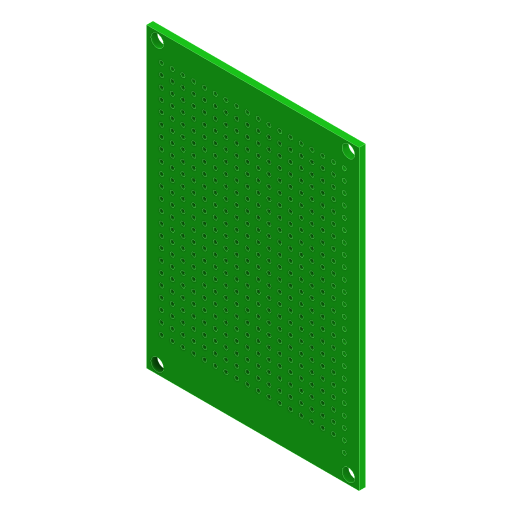
# Autodesk Inventor part: Плата главная
Saved by Autodesk Inventor 2023 (Build 270158000, 158)
## iProperties
Created: 2023-01-03
Part Number: Плата главная
Material: Типовые
Document SubType Name: Modeling
Designer: Admin
Density: 1 g/cm^3
Appearance: По умолчанию
Author: Admin
Autodesk Inventor part; units mm, degrees
ref_plane "YZ Plane" through (0, 0, 0) normal (1, 0, 0) x (0, 1, 0)
ref_plane "XZ Plane" through (0, 0, 0) normal (0, 1, 0) x (-1, 0, 0)
ref_plane "XY Plane" through (0, 0, 0) normal (0, 0, 1) x (1, 0, 0)
sketch "Эскиз1" plane through (0, 0, 0) normal (0, 0, 1) x (1, 0, 0)
  line L0 (25, 35) -> (-25, 35)
  line L1 (-25, 35) -> (-25, -35)
  line L2 (-25, -35) -> (25, -35)
  line L3 (25, -35) -> (25, 35)
  circle A0 centre (22.5, 33) radius 1.5
  circle A1 centre (-22.5, 33) radius 1.5
  circle A2 centre (-22.5, -33) radius 1.5
  circle A3 centre (22.5, -33) radius 1.5
  line L4 (0, 0) -> (8.4317, 0) construction
  line L5 (8.4317, 0) -> (0, 0) construction
  line L6 (0, 0) -> (0, -9.142) construction
  circle A4 centre (21.505, -28.98) radius 0.5
  circle A5 centre (21.505, -26.46) radius 0.5
  circle A6 centre (21.505, -23.94) radius 0.5
  circle A7 centre (21.505, -21.42) radius 0.5
  circle A8 centre (21.505, -18.9) radius 0.5
  circle A9 centre (21.505, -16.38) radius 0.5
  circle A10 centre (21.505, -13.86) radius 0.5
  circle A11 centre (21.505, -11.34) radius 0.5
  circle A12 centre (21.505, -8.82) radius 0.5
  circle A13 centre (21.505, -6.3) radius 0.5
  circle A14 centre (21.505, -3.78) radius 0.5
  circle A15 centre (21.505, -1.26) radius 0.5
  circle A16 centre (21.505, 1.26) radius 0.5
  circle A17 centre (21.505, 3.78) radius 0.5
  circle A18 centre (21.505, 6.3) radius 0.5
  circle A19 centre (21.505, 8.82) radius 0.5
  circle A20 centre (21.505, 11.34) radius 0.5
  circle A21 centre (21.505, 13.86) radius 0.5
  circle A22 centre (21.505, 16.38) radius 0.5
  circle A23 centre (21.505, 18.9) radius 0.5
  circle A24 centre (21.505, 21.42) radius 0.5
  circle A25 centre (21.505, 23.94) radius 0.5
  circle A26 centre (21.505, 26.46) radius 0.5
  circle A27 centre (21.505, 28.98) radius 0.5
  line L7 (25, 0) -> (23.0544, 0) construction
  circle A28 centre (18.975, -26.46) radius 0.5
  circle A29 centre (18.975, -23.94) radius 0.5
  circle A30 centre (18.975, -21.42) radius 0.5
  circle A31 centre (18.975, -18.9) radius 0.5
  circle A32 centre (18.975, -16.38) radius 0.5
  circle A33 centre (18.975, -13.86) radius 0.5
  circle A34 centre (18.975, -11.34) radius 0.5
  circle A35 centre (18.975, -8.82) radius 0.5
  circle A36 centre (18.975, -6.3) radius 0.5
  circle A37 centre (18.975, -3.78) radius 0.5
  circle A38 centre (18.975, -1.26) radius 0.5
  circle A39 centre (18.975, 1.26) radius 0.5
  circle A40 centre (18.975, 3.78) radius 0.5
  circle A41 centre (18.975, 6.3) radius 0.5
  circle A42 centre (18.975, 8.82) radius 0.5
  circle A43 centre (18.975, 11.34) radius 0.5
  circle A44 centre (18.975, 13.86) radius 0.5
  circle A45 centre (18.975, 16.38) radius 0.5
  circle A46 centre (18.975, 18.9) radius 0.5
  circle A47 centre (18.975, 21.42) radius 0.5
  circle A48 centre (18.975, 23.94) radius 0.5
  circle A49 centre (18.975, 26.46) radius 0.5
  circle A50 centre (18.975, 28.98) radius 0.5
  circle A51 centre (16.445, -26.46) radius 0.5
  circle A52 centre (16.445, -23.94) radius 0.5
  circle A53 centre (16.445, -21.42) radius 0.5
  circle A54 centre (16.445, -18.9) radius 0.5
  circle A55 centre (16.445, -16.38) radius 0.5
  circle A56 centre (16.445, -13.86) radius 0.5
  circle A57 centre (16.445, -11.34) radius 0.5
  circle A58 centre (16.445, -8.82) radius 0.5
  circle A59 centre (16.445, -6.3) radius 0.5
  circle A60 centre (16.445, -3.78) radius 0.5
  circle A61 centre (16.445, -1.26) radius 0.5
  circle A62 centre (16.445, 1.26) radius 0.5
  circle A63 centre (16.445, 3.78) radius 0.5
  circle A64 centre (16.445, 6.3) radius 0.5
  circle A65 centre (16.445, 8.82) radius 0.5
  circle A66 centre (16.445, 11.34) radius 0.5
  circle A67 centre (16.445, 13.86) radius 0.5
  circle A68 centre (16.445, 16.38) radius 0.5
  circle A69 centre (16.445, 18.9) radius 0.5
  circle A70 centre (16.445, 21.42) radius 0.5
  circle A71 centre (16.445, 23.94) radius 0.5
  circle A72 centre (16.445, 26.46) radius 0.5
  circle A73 centre (16.445, 28.98) radius 0.5
  circle A74 centre (13.915, -26.46) radius 0.5
  circle A75 centre (13.915, -23.94) radius 0.5
  circle A76 centre (13.915, -21.42) radius 0.5
  circle A77 centre (13.915, -18.9) radius 0.5
  circle A78 centre (13.915, -16.38) radius 0.5
  circle A79 centre (13.915, -13.86) radius 0.5
  circle A80 centre (13.915, -11.34) radius 0.5
  circle A81 centre (13.915, -8.82) radius 0.5
  circle A82 centre (13.915, -6.3) radius 0.5
  circle A83 centre (13.915, -3.78) radius 0.5
  circle A84 centre (13.915, -1.26) radius 0.5
  circle A85 centre (13.915, 1.26) radius 0.5
  circle A86 centre (13.915, 3.78) radius 0.5
  circle A87 centre (13.915, 6.3) radius 0.5
  circle A88 centre (13.915, 8.82) radius 0.5
  circle A89 centre (13.915, 11.34) radius 0.5
  circle A90 centre (13.915, 13.86) radius 0.5
  circle A91 centre (13.915, 16.38) radius 0.5
  circle A92 centre (13.915, 18.9) radius 0.5
  circle A93 centre (13.915, 21.42) radius 0.5
  circle A94 centre (13.915, 23.94) radius 0.5
  circle A95 centre (13.915, 26.46) radius 0.5
  circle A96 centre (13.915, 28.98) radius 0.5
  circle A97 centre (11.385, -26.46) radius 0.5
  circle A98 centre (11.385, -23.94) radius 0.5
  circle A99 centre (11.385, -21.42) radius 0.5
  circle A100 centre (11.385, -18.9) radius 0.5
  circle A101 centre (11.385, -16.38) radius 0.5
  circle A102 centre (11.385, -13.86) radius 0.5
  circle A103 centre (11.385, -11.34) radius 0.5
  circle A104 centre (11.385, -8.82) radius 0.5
  circle A105 centre (11.385, -6.3) radius 0.5
  circle A106 centre (11.385, -3.78) radius 0.5
  circle A107 centre (11.385, -1.26) radius 0.5
  circle A108 centre (11.385, 1.26) radius 0.5
  circle A109 centre (11.385, 3.78) radius 0.5
  circle A110 centre (11.385, 6.3) radius 0.5
  circle A111 centre (11.385, 8.82) radius 0.5
  circle A112 centre (11.385, 11.34) radius 0.5
  circle A113 centre (11.385, 13.86) radius 0.5
  circle A114 centre (11.385, 16.38) radius 0.5
  circle A115 centre (11.385, 18.9) radius 0.5
  circle A116 centre (11.385, 21.42) radius 0.5
  circle A117 centre (11.385, 23.94) radius 0.5
  circle A118 centre (11.385, 26.46) radius 0.5
  circle A119 centre (11.385, 28.98) radius 0.5
  circle A120 centre (8.855, -26.46) radius 0.5
  circle A121 centre (8.855, -23.94) radius 0.5
  circle A122 centre (8.855, -21.42) radius 0.5
  circle A123 centre (8.855, -18.9) radius 0.5
  circle A124 centre (8.855, -16.38) radius 0.5
  circle A125 centre (8.855, -13.86) radius 0.5
  circle A126 centre (8.855, -11.34) radius 0.5
  circle A127 centre (8.855, -8.82) radius 0.5
  circle A128 centre (8.855, -6.3) radius 0.5
  circle A129 centre (8.855, -3.78) radius 0.5
  circle A130 centre (8.855, -1.26) radius 0.5
  circle A131 centre (8.855, 1.26) radius 0.5
  circle A132 centre (8.855, 3.78) radius 0.5
  circle A133 centre (8.855, 6.3) radius 0.5
  circle A134 centre (8.855, 8.82) radius 0.5
  circle A135 centre (8.855, 11.34) radius 0.5
  circle A136 centre (8.855, 13.86) radius 0.5
  circle A137 centre (8.855, 16.38) radius 0.5
  circle A138 centre (8.855, 18.9) radius 0.5
  circle A139 centre (8.855, 21.42) radius 0.5
  circle A140 centre (8.855, 23.94) radius 0.5
  circle A141 centre (8.855, 26.46) radius 0.5
  circle A142 centre (8.855, 28.98) radius 0.5
  circle A143 centre (6.325, -26.46) radius 0.5
  circle A144 centre (6.325, -23.94) radius 0.5
  circle A145 centre (6.325, -21.42) radius 0.5
  circle A146 centre (6.325, -18.9) radius 0.5
  circle A147 centre (6.325, -16.38) radius 0.5
  circle A148 centre (6.325, -13.86) radius 0.5
  circle A149 centre (6.325, -11.34) radius 0.5
  circle A150 centre (6.325, -8.82) radius 0.5
  circle A151 centre (6.325, -6.3) radius 0.5
  circle A152 centre (6.325, -3.78) radius 0.5
  circle A153 centre (6.325, -1.26) radius 0.5
  circle A154 centre (6.325, 1.26) radius 0.5
  circle A155 centre (6.325, 3.78) radius 0.5
  circle A156 centre (6.325, 6.3) radius 0.5
  circle A157 centre (6.325, 8.82) radius 0.5
  circle A158 centre (6.325, 11.34) radius 0.5
  circle A159 centre (6.325, 13.86) radius 0.5
  circle A160 centre (6.325, 16.38) radius 0.5
  circle A161 centre (6.325, 18.9) radius 0.5
  circle A162 centre (6.325, 21.42) radius 0.5
  circle A163 centre (6.325, 23.94) radius 0.5
  circle A164 centre (6.325, 26.46) radius 0.5
  circle A165 centre (6.325, 28.98) radius 0.5
  circle A166 centre (3.795, -26.46) radius 0.5
  circle A167 centre (3.795, -23.94) radius 0.5
  circle A168 centre (3.795, -21.42) radius 0.5
  circle A169 centre (3.795, -18.9) radius 0.5
  circle A170 centre (3.795, -16.38) radius 0.5
  circle A171 centre (3.795, -13.86) radius 0.5
  circle A172 centre (3.795, -11.34) radius 0.5
  circle A173 centre (3.795, -8.82) radius 0.5
  circle A174 centre (3.795, -6.3) radius 0.5
  circle A175 centre (3.795, -3.78) radius 0.5
  circle A176 centre (3.795, -1.26) radius 0.5
  circle A177 centre (3.795, 1.26) radius 0.5
  circle A178 centre (3.795, 3.78) radius 0.5
  circle A179 centre (3.795, 6.3) radius 0.5
  circle A180 centre (3.795, 8.82) radius 0.5
  circle A181 centre (3.795, 11.34) radius 0.5
  circle A182 centre (3.795, 13.86) radius 0.5
  circle A183 centre (3.795, 16.38) radius 0.5
  circle A184 centre (3.795, 18.9) radius 0.5
  circle A185 centre (3.795, 21.42) radius 0.5
  circle A186 centre (3.795, 23.94) radius 0.5
  circle A187 centre (3.795, 26.46) radius 0.5
  circle A188 centre (3.795, 28.98) radius 0.5
  circle A189 centre (1.265, -26.46) radius 0.5
  circle A190 centre (1.265, -23.94) radius 0.5
  circle A191 centre (1.265, -21.42) radius 0.5
  circle A192 centre (1.265, -18.9) radius 0.5
  circle A193 centre (1.265, -16.38) radius 0.5
  circle A194 centre (1.265, -13.86) radius 0.5
  circle A195 centre (1.265, -11.34) radius 0.5
  circle A196 centre (1.265, -8.82) radius 0.5
  circle A197 centre (1.265, -6.3) radius 0.5
  circle A198 centre (1.265, -3.78) radius 0.5
  circle A199 centre (1.265, -1.26) radius 0.5
  circle A200 centre (1.265, 1.26) radius 0.5
  circle A201 centre (1.265, 3.78) radius 0.5
  circle A202 centre (1.265, 6.3) radius 0.5
  circle A203 centre (1.265, 8.82) radius 0.5
  circle A204 centre (1.265, 11.34) radius 0.5
  circle A205 centre (1.265, 13.86) radius 0.5
  circle A206 centre (1.265, 16.38) radius 0.5
  circle A207 centre (1.265, 18.9) radius 0.5
  circle A208 centre (1.265, 21.42) radius 0.5
  circle A209 centre (1.265, 23.94) radius 0.5
  circle A210 centre (1.265, 26.46) radius 0.5
  circle A211 centre (1.265, 28.98) radius 0.5
  circle A212 centre (-1.265, -26.46) radius 0.5
  circle A213 centre (-1.265, -23.94) radius 0.5
  circle A214 centre (-1.265, -21.42) radius 0.5
  circle A215 centre (-1.265, -18.9) radius 0.5
  circle A216 centre (-1.265, -16.38) radius 0.5
  circle A217 centre (-1.265, -13.86) radius 0.5
  circle A218 centre (-1.265, -11.34) radius 0.5
  circle A219 centre (-1.265, -8.82) radius 0.5
  circle A220 centre (-1.265, -6.3) radius 0.5
  circle A221 centre (-1.265, -3.78) radius 0.5
  circle A222 centre (-1.265, -1.26) radius 0.5
  circle A223 centre (-1.265, 1.26) radius 0.5
  circle A224 centre (-1.265, 3.78) radius 0.5
  circle A225 centre (-1.265, 6.3) radius 0.5
  circle A226 centre (-1.265, 8.82) radius 0.5
  circle A227 centre (-1.265, 11.34) radius 0.5
  circle A228 centre (-1.265, 13.86) radius 0.5
  circle A229 centre (-1.265, 16.38) radius 0.5
  circle A230 centre (-1.265, 18.9) radius 0.5
  circle A231 centre (-1.265, 21.42) radius 0.5
  circle A232 centre (-1.265, 23.94) radius 0.5
  circle A233 centre (-1.265, 26.46) radius 0.5
  circle A234 centre (-1.265, 28.98) radius 0.5
  circle A235 centre (-3.795, -26.46) radius 0.5
  circle A236 centre (-3.795, -23.94) radius 0.5
  circle A237 centre (-3.795, -21.42) radius 0.5
  circle A238 centre (-3.795, -18.9) radius 0.5
  circle A239 centre (-3.795, -16.38) radius 0.5
  circle A240 centre (-3.795, -13.86) radius 0.5
  circle A241 centre (-3.795, -11.34) radius 0.5
  circle A242 centre (-3.795, -8.82) radius 0.5
  circle A243 centre (-3.795, -6.3) radius 0.5
  circle A244 centre (-3.795, -3.78) radius 0.5
  circle A245 centre (-3.795, -1.26) radius 0.5
  circle A246 centre (-3.795, 1.26) radius 0.5
  circle A247 centre (-3.795, 3.78) radius 0.5
  circle A248 centre (-3.795, 6.3) radius 0.5
  circle A249 centre (-3.795, 8.82) radius 0.5
  circle A250 centre (-3.795, 11.34) radius 0.5
  circle A251 centre (-3.795, 13.86) radius 0.5
  circle A252 centre (-3.795, 16.38) radius 0.5
  circle A253 centre (-3.795, 18.9) radius 0.5
  circle A254 centre (-3.795, 21.42) radius 0.5
  circle A255 centre (-3.795, 23.94) radius 0.5
  circle A256 centre (-3.795, 26.46) radius 0.5
  circle A257 centre (-3.795, 28.98) radius 0.5
  circle A258 centre (-6.325, -26.46) radius 0.5
  circle A259 centre (-6.325, -23.94) radius 0.5
  circle A260 centre (-6.325, -21.42) radius 0.5
  circle A261 centre (-6.325, -18.9) radius 0.5
  circle A262 centre (-6.325, -16.38) radius 0.5
  circle A263 centre (-6.325, -13.86) radius 0.5
  circle A264 centre (-6.325, -11.34) radius 0.5
  circle A265 centre (-6.325, -8.82) radius 0.5
  circle A266 centre (-6.325, -6.3) radius 0.5
  circle A267 centre (-6.325, -3.78) radius 0.5
  circle A268 centre (-6.325, -1.26) radius 0.5
  circle A269 centre (-6.325, 1.26) radius 0.5
  circle A270 centre (-6.325, 3.78) radius 0.5
  circle A271 centre (-6.325, 6.3) radius 0.5
  circle A272 centre (-6.325, 8.82) radius 0.5
  circle A273 centre (-6.325, 11.34) radius 0.5
  circle A274 centre (-6.325, 13.86) radius 0.5
  circle A275 centre (-6.325, 16.38) radius 0.5
  circle A276 centre (-6.325, 18.9) radius 0.5
  circle A277 centre (-6.325, 21.42) radius 0.5
  circle A278 centre (-6.325, 23.94) radius 0.5
  circle A279 centre (-6.325, 26.46) radius 0.5
  circle A280 centre (-6.325, 28.98) radius 0.5
  circle A281 centre (-8.855, -26.46) radius 0.5
  circle A282 centre (-8.855, -23.94) radius 0.5
  circle A283 centre (-8.855, -21.42) radius 0.5
  circle A284 centre (-8.855, -18.9) radius 0.5
  circle A285 centre (-8.855, -16.38) radius 0.5
  circle A286 centre (-8.855, -13.86) radius 0.5
  circle A287 centre (-8.855, -11.34) radius 0.5
  circle A288 centre (-8.855, -8.82) radius 0.5
  circle A289 centre (-8.855, -6.3) radius 0.5
  circle A290 centre (-8.855, -3.78) radius 0.5
  circle A291 centre (-8.855, -1.26) radius 0.5
  circle A292 centre (-8.855, 1.26) radius 0.5
  circle A293 centre (-8.855, 3.78) radius 0.5
  circle A294 centre (-8.855, 6.3) radius 0.5
  circle A295 centre (-8.855, 8.82) radius 0.5
  circle A296 centre (-8.855, 11.34) radius 0.5
  circle A297 centre (-8.855, 13.86) radius 0.5
  circle A298 centre (-8.855, 16.38) radius 0.5
  circle A299 centre (-8.855, 18.9) radius 0.5
  circle A300 centre (-8.855, 21.42) radius 0.5
  circle A301 centre (-8.855, 23.94) radius 0.5
  circle A302 centre (-8.855, 26.46) radius 0.5
  circle A303 centre (-8.855, 28.98) radius 0.5
  circle A304 centre (-11.385, -26.46) radius 0.5
  circle A305 centre (-11.385, -23.94) radius 0.5
  circle A306 centre (-11.385, -21.42) radius 0.5
  circle A307 centre (-11.385, -18.9) radius 0.5
  circle A308 centre (-11.385, -16.38) radius 0.5
  circle A309 centre (-11.385, -13.86) radius 0.5
  circle A310 centre (-11.385, -11.34) radius 0.5
  circle A311 centre (-11.385, -8.82) radius 0.5
  circle A312 centre (-11.385, -6.3) radius 0.5
  circle A313 centre (-11.385, -3.78) radius 0.5
  circle A314 centre (-11.385, -1.26) radius 0.5
  circle A315 centre (-11.385, 1.26) radius 0.5
  circle A316 centre (-11.385, 3.78) radius 0.5
  circle A317 centre (-11.385, 6.3) radius 0.5
  circle A318 centre (-11.385, 8.82) radius 0.5
  circle A319 centre (-11.385, 11.34) radius 0.5
  circle A320 centre (-11.385, 13.86) radius 0.5
  circle A321 centre (-11.385, 16.38) radius 0.5
  circle A322 centre (-11.385, 18.9) radius 0.5
  circle A323 centre (-11.385, 21.42) radius 0.5
  circle A324 centre (-11.385, 23.94) radius 0.5
  circle A325 centre (-11.385, 26.46) radius 0.5
  circle A326 centre (-11.385, 28.98) radius 0.5
  circle A327 centre (-13.915, -26.46) radius 0.5
  circle A328 centre (-13.915, -23.94) radius 0.5
  circle A329 centre (-13.915, -21.42) radius 0.5
  circle A330 centre (-13.915, -18.9) radius 0.5
  circle A331 centre (-13.915, -16.38) radius 0.5
  circle A332 centre (-13.915, -13.86) radius 0.5
  circle A333 centre (-13.915, -11.34) radius 0.5
  circle A334 centre (-13.915, -8.82) radius 0.5
  circle A335 centre (-13.915, -6.3) radius 0.5
  circle A336 centre (-13.915, -3.78) radius 0.5
  circle A337 centre (-13.915, -1.26) radius 0.5
  circle A338 centre (-13.915, 1.26) radius 0.5
  circle A339 centre (-13.915, 3.78) radius 0.5
  circle A340 centre (-13.915, 6.3) radius 0.5
  circle A341 centre (-13.915, 8.82) radius 0.5
  circle A342 centre (-13.915, 11.34) radius 0.5
  circle A343 centre (-13.915, 13.86) radius 0.5
  circle A344 centre (-13.915, 16.38) radius 0.5
  circle A345 centre (-13.915, 18.9) radius 0.5
  circle A346 centre (-13.915, 21.42) radius 0.5
  circle A347 centre (-13.915, 23.94) radius 0.5
  circle A348 centre (-13.915, 26.46) radius 0.5
  circle A349 centre (-13.915, 28.98) radius 0.5
  circle A350 centre (-16.445, -26.46) radius 0.5
  circle A351 centre (-16.445, -23.94) radius 0.5
  circle A352 centre (-16.445, -21.42) radius 0.5
  circle A353 centre (-16.445, -18.9) radius 0.5
  circle A354 centre (-16.445, -16.38) radius 0.5
  circle A355 centre (-16.445, -13.86) radius 0.5
  circle A356 centre (-16.445, -11.34) radius 0.5
  circle A357 centre (-16.445, -8.82) radius 0.5
  circle A358 centre (-16.445, -6.3) radius 0.5
  circle A359 centre (-16.445, -3.78) radius 0.5
  circle A360 centre (-16.445, -1.26) radius 0.5
  circle A361 centre (-16.445, 1.26) radius 0.5
  circle A362 centre (-16.445, 3.78) radius 0.5
  circle A363 centre (-16.445, 6.3) radius 0.5
  circle A364 centre (-16.445, 8.82) radius 0.5
  circle A365 centre (-16.445, 11.34) radius 0.5
  circle A366 centre (-16.445, 13.86) radius 0.5
  circle A367 centre (-16.445, 16.38) radius 0.5
  circle A368 centre (-16.445, 18.9) radius 0.5
  circle A369 centre (-16.445, 21.42) radius 0.5
  circle A370 centre (-16.445, 23.94) radius 0.5
  circle A371 centre (-16.445, 26.46) radius 0.5
  circle A372 centre (-16.445, 28.98) radius 0.5
  circle A373 centre (-18.975, -26.46) radius 0.5
  circle A374 centre (-18.975, -23.94) radius 0.5
  circle A375 centre (-18.975, -21.42) radius 0.5
  circle A376 centre (-18.975, -18.9) radius 0.5
  circle A377 centre (-18.975, -16.38) radius 0.5
  circle A378 centre (-18.975, -13.86) radius 0.5
  circle A379 centre (-18.975, -11.34) radius 0.5
  circle A380 centre (-18.975, -8.82) radius 0.5
  circle A381 centre (-18.975, -6.3) radius 0.5
  circle A382 centre (-18.975, -3.78) radius 0.5
  circle A383 centre (-18.975, -1.26) radius 0.5
  circle A384 centre (-18.975, 1.26) radius 0.5
  circle A385 centre (-18.975, 3.78) radius 0.5
  circle A386 centre (-18.975, 6.3) radius 0.5
  circle A387 centre (-18.975, 8.82) radius 0.5
  circle A388 centre (-18.975, 11.34) radius 0.5
  circle A389 centre (-18.975, 13.86) radius 0.5
  circle A390 centre (-18.975, 16.38) radius 0.5
  circle A391 centre (-18.975, 18.9) radius 0.5
  circle A392 centre (-18.975, 21.42) radius 0.5
  circle A393 centre (-18.975, 23.94) radius 0.5
  circle A394 centre (-18.975, 26.46) radius 0.5
  circle A395 centre (-18.975, 28.98) radius 0.5
  circle A396 centre (-21.505, -26.46) radius 0.5
  circle A397 centre (-21.505, -23.94) radius 0.5
  circle A398 centre (-21.505, -21.42) radius 0.5
  circle A399 centre (-21.505, -18.9) radius 0.5
  circle A400 centre (-21.505, -16.38) radius 0.5
  circle A401 centre (-21.505, -13.86) radius 0.5
  circle A402 centre (-21.505, -11.34) radius 0.5
  circle A403 centre (-21.505, -8.82) radius 0.5
  circle A404 centre (-21.505, -6.3) radius 0.5
  circle A405 centre (-21.505, -3.78) radius 0.5
  circle A406 centre (-21.505, -1.26) radius 0.5
  circle A407 centre (-21.505, 1.26) radius 0.5
  circle A408 centre (-21.505, 3.78) radius 0.5
  circle A409 centre (-21.505, 6.3) radius 0.5
  circle A410 centre (-21.505, 8.82) radius 0.5
  circle A411 centre (-21.505, 11.34) radius 0.5
  circle A412 centre (-21.505, 13.86) radius 0.5
  circle A413 centre (-21.505, 16.38) radius 0.5
  circle A414 centre (-21.505, 18.9) radius 0.5
  circle A415 centre (-21.505, 21.42) radius 0.5
  circle A416 centre (-21.505, 23.94) radius 0.5
  circle A417 centre (-21.505, 26.46) radius 0.5
  circle A418 centre (-21.505, 28.98) radius 0.5
  line L8 (0, 35) -> (0, 33) construction
  point P0 (-25, 0)
  point P1 (0, -35)
  dimension "d1" = 70
  dimension "d2" = 50
  dimension "d3" = 42
  dimension "d4" = 63
  dimension "d5" = 3
  dimension "d16" = 1
  dimension "d19" = 2.52
  dimension "d27" = 2.53
  constraints: 419 centre point, 18 end point, 4 horizontal, 4 midpoint, 3 equal length, 3 equal radius, 3 horizontal alignment, 3 vertical, 3 vertical alignment, 1 coincident, 1 perpendicular, 832 other
  measures "d1" distance of L3.start L3.end
  measures "d2" distance of L3.end L0.end
  measures "d5" diameter of A2
  measures "d16" diameter of A4
  measures "d19" distance of A4.centre A5.centre
  measures "d27" distance of A6.centre A29.centre
extrude "Выдавливание1" add sketch "Эскиз1" along normal blind 1.5
